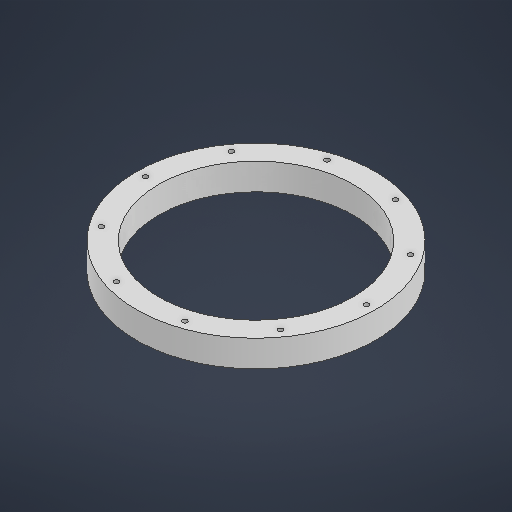
# Autodesk Inventor part: Cylinder Bottom
Saved by Autodesk Inventor 2025 (Build 290162000, 162)
## iProperties
Created: 2024-04-29
Part Number: Cylinder Bottom
Material: Generic
Document SubType Name: Modeling
Designer: Thienan Hoang
Density: 1 g/cm^3
Appearance: Default
Author: Thienan Hoang
Autodesk Inventor part; units mm, degrees
ref_plane "YZ Plane" through (0, 0, 0) normal (1, 0, 0) x (0, 1, 0)
ref_plane "XZ Plane" through (0, 0, 0) normal (0, 1, 0) x (-1, 0, 0)
ref_plane "XY Plane" through (0, 0, 0) normal (0, 0, 1) x (1, 0, 0)
sketch "Sketch1" plane through (0, 0, 0) normal (0, 1, 0) x (-1, 0, 0)
  circle A0 centre (0, 0) radius 135
  circle A1 centre (0, 0) radius 110
  dimension "d0" = 270
  dimension "d1" = 220
  constraints: 2 centre point, 2 coincident
  measures "d0" diameter of A0
  measures "d1" diameter of A1
extrude "Extrusion1" add sketch "Sketch1" along normal blind 30
sketch "Sketch3" plane through (0, 30, 0) normal (0, 1, 0) x (1, 0, 0)
  circle A0 centre (0, 0) radius 125
  circle A1 centre (-125, 0) radius 2
  circle A2 centre (-101.1271, -73.4732) radius 2
  circle A3 centre (-38.6271, -118.8821) radius 2
  circle A4 centre (38.6271, -118.8821) radius 2
  circle A5 centre (101.1271, -73.4732) radius 2
  circle A6 centre (125, 0) radius 2
  circle A7 centre (101.1271, 73.4732) radius 2
  circle A8 centre (38.6271, 118.8821) radius 2
  circle A9 centre (-38.6271, 118.8821) radius 2
  circle A10 centre (-101.1271, 73.4732) radius 2
  dimension "d8" = 250
  dimension "d9" = 4
  dimension "d12" = 360
  constraints: 10 centre point, 1 coincident, 1 horizontal alignment, 23 other
  measures "d9" diameter of A1
hole "Hole1" at (101.1271, 30, 73.4732) at (125, 30, 0) at (101.1271, 30, -73.4732) at (38.6271, 30, -118.8821) at (-38.6271, 30, -118.8821) at (-101.1271, 30, -73.4732) at (-125, 30, 0) at (-101.1271, 30, 73.4732) at (-38.6271, 30, 118.8821) at (38.6271, 30, 118.8821) direction (0, -1, 0) diameter 5.5 end through all
sketch "Sketch8" plane through (0, 30, 0) normal (0, 1, 0) x (1, 0, 0)
  circle A0 centre (0, 0) radius 110
  circle A1 centre (0, 0) radius 62.5
  dimension "d36" = 125
  dimension "d41" = 220
  constraints: 2 centre point, 2 coincident
  measures "d36" diameter of A1
  measures "d41" diameter of A0
extrude "Extrusion7" [suppressed]
sketch "Sketch9" plane through (0, 30, 0) normal (0, 1, 0) x (1, 0, 0)
  circle A0 centre (0, 0) radius 110
  constraints: 1 centre point, 1 coincident
extrude "Extrusion8" [suppressed]
sketch "Sketch10" plane through (0, 25, 0) normal (0, 1, 0) x (1, 0, 0)
  circle A0 centre (0, 0) radius 65
  circle A1 centre (0, 0) radius 62.5
  dimension "d42" = 130
  constraints: 2 centre point, 2 coincident
  measures "d42" diameter of A0
extrude "Extrusion9" [suppressed]
sketch "Sketch11" plane through (0, 25, 0) normal (0, 1, 0) x (1, 0, 0)
  circle A0 centre (0, 0) radius 75
  circle A1 centre (0, 0) radius 65 projected
  circle A2 centre (0, 0) radius 76.5
  dimension "d45" = 150
  dimension "d46" = 153
  constraints: 2 centre point, 2 coincident
  measures "d45" diameter of A0
  measures "d46" diameter of A2
extrude "Extrusion10" [suppressed]
sketch "Sketch12" plane through (0, 25, 0) normal (0, 1, 0) x (1, 0, 0)
  circle A0 centre (0, 0) radius 85
  circle A1 centre (0, -85) radius 2.75
  circle A2 centre (73.6122, -42.5) radius 2.75
  circle A3 centre (73.6122, 42.5) radius 2.75
  circle A4 centre (0, 85) radius 2.75
  circle A5 centre (-73.6122, 42.5) radius 2.75
  circle A6 centre (-73.6122, -42.5) radius 2.75
  dimension "d49" = 170
  dimension "d55" = 5.5
  dimension "d58" = 360
  constraints: 6 centre point, 1 coincident, 1 vertical alignment, 15 other
  measures "d55" diameter of A1
extrude "Extrusion11" [suppressed]
body "Solid1"
